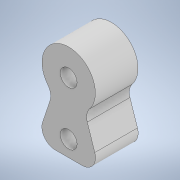
# Autodesk Inventor part: Part2
Saved by Autodesk Inventor 2022 (Build 260153000, 153)
## iProperties
Created: 2021-04-05
Part Number: Part2
Material: Generic
Document SubType Name: Modeling
Designer: chris
Density: 1 g/cm^3
Appearance: Default
Author: chris
Autodesk Inventor part; units mm, degrees
ref_plane "YZ Plane" through (0, 0, 0) normal (1, 0, 0) x (0, 1, 0)
ref_plane "XZ Plane" through (0, 0, 0) normal (0, 1, 0) x (-1, 0, 0)
ref_plane "XY Plane" through (0, 0, 0) normal (0, 0, 1) x (1, 0, 0)
sketch "Sketch1" plane through (0, 0, 0) normal (0, 0, 1) x (1, 0, 0)
  circle A0 centre (0, 0) radius 1.0033
  circle A1 centre (0, 0) radius 3.175
  line L0 (-1.905, -8.255) -> (1.905, -8.255)
  line L1 (1.905, -8.255) -> (1.905, -2.54)
  line L2 (-1.905, -8.255) -> (-1.905, -2.54)
  circle A2 centre (0, -6.35) radius 1.0033
  line L3 (1.905, -8.255) -> (3.81, -8.255)
  line L4 (3.81, -8.255) -> (1.905, -2.54)
  line L5 (-1.905, -8.255) -> (-3.81, -8.255)
  line L6 (-3.81, -8.255) -> (-1.905, -2.54)
  point P0 (0, -8.255)
  dimension "d0" = 2.0066
  dimension "d1" = 6.35
  dimension "d2" = 3.81
  dimension "d3" = 2.0066
  dimension "d4" = 5.715
  dimension "d5" = 1.905
  dimension "d10" = 1.905
  dimension "d11" = 1.905
  constraints: 14 end point, 3 centre point, 2 coincident, 2 horizontal, 2 point on circle, 1 midpoint, 1 parallel, 1 point on line, 1 vertical, 1 vertical alignment
  measures "d0" diameter of A0
  measures "d1" diameter of A1
  measures "d2" distance of L0.start L0.end
  measures "d3" diameter of A2
  measures "d4" distance of L0.end L1.end
  measures "d5" distance from line of L0 A2.centre
  measures "d10" distance of L0.end L3.end
  measures "d11" distance of L0.start L5.end
extrude "Extrusion1" add sketch "Sketch1" along normal blind 5.08 contours A1 | A1 L1 L0 L2
extrude "Extrusion3" add sketch "Sketch1" along normal blind 5.08 contours L2 L5 L6 | L4 L3 L1
fillet "Fillet1" radius 1.5875 4 edges at (3.81, -8.255, 2.54) (-3.81, -8.255, 2.54) (1.905, -2.54, 2.54) (-1.905, -2.54, 2.54)
body "Solid1"
